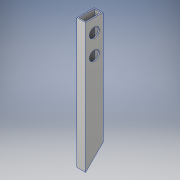
# Autodesk Inventor part: StorageSupport.ver1-1111-2020
Saved by Autodesk Inventor 2018 (Build 220112000, 112)
## iProperties
Created: 2020-01-25
Part Number: StorageSupport.ver1-1111-2020
Material: Aluminum 6061
Document SubType Name: Modeling
Designer: JMHal
Density: 2.7 g/cm^3
Appearance: Aluminum - Flat
Author: JMHal
Autodesk Inventor part; units mm, degrees
ref_plane "YZ Plane" through (0, 0, 0) normal (1, 0, 0) x (0, 1, 0)
ref_plane "XZ Plane" through (0, 0, 0) normal (0, 1, 0) x (-1, 0, 0)
ref_plane "XY Plane" through (0, 0, 0) normal (0, 0, 1) x (1, 0, 0)
sketch "Sketch1" plane through (0, 0, 0) normal (0, 1, 0) x (-1, 0, 0)
  line L0 (0, 0) -> (25.4, 0)
  line L1 (25.4, 0) -> (25.4, -50.8)
  line L2 (25.4, -50.8) -> (0, -50.8)
  line L3 (0, -50.8) -> (0, 0)
  line L4 (22.225, -3.175) -> (3.175, -3.175)
  line L5 (3.175, -3.175) -> (3.175, -47.625)
  line L6 (3.175, -47.625) -> (22.225, -47.625)
  line L7 (22.225, -47.625) -> (22.225, -3.175)
  dimension "d0" = 25.4
  dimension "d1" = 50.8
  dimension "d2" = 3.175
  constraints: 16 end point, 4 parallel, 2 perpendicular, 1 horizontal, 3 other
  measures "d0" distance of L1.end L2.end
  measures "d1" distance of L0.end L1.end
  measures "d2" distance between parallel lines of L0 L4
extrude "Extrusion1" add sketch "Sketch1" along normal blind 106.553
sketch "Sketch3" plane through (0, 0, 0) normal (1, 0, 0) x (0, 0, -1)
  line L0 (50.8, 0) -> (0, 0) projected
  line L1 (50.8, 0) -> (50.8, 106.553) projected
  line L2 (0, 106.553) -> (50.8, 106.553) projected
  line L3 (0, 0) -> (0, 106.553) projected
  point P0 (25.4, 68.453)
  dimension "d19" = 38.1
  measures "d19" distance from line of L2 point (25.4, 68.453)
hole "Hole2" at (0, 68.453, -25.4) direction (-1, 0, 0) diameter 28.575 end through all
sketch "Sketch4" plane through (0, 0, 0) normal (0, -1, 0) x (1, 0, 0)
  line L0 (-22.225, -47.625) -> (-22.225, -3.175) projected
  line L1 (-22.225, -3.175) -> (-3.175, -3.175) projected
  line L2 (-3.175, -3.175) -> (-3.175, -47.625) projected
  line L3 (-3.175, -47.625) -> (-22.225, -47.625) projected
  line L4 (0, 0) -> (-25.4, 0) projected
  line L5 (-25.4, 0) -> (-25.4, -50.8) projected
  line L6 (-25.4, -50.8) -> (0, -50.8) projected
  line L7 (0, -50.8) -> (0, 0) projected
extrude "Extrusion2" add sketch "Sketch4" along normal blind 254
sketch "Sketch5" plane through (0, 106.553, 0) normal (1, 0, 0) x (0, 0, -1)
  circle A0 centre (25.4, -38.1) radius 14.2875 projected
  line L0 (50.8, 0) -> (50.8, -360.553) projected
  line L1 (0, 0) -> (50.8, 0) projected
  line L2 (0, -360.553) -> (0, 0) projected
  line L3 (50.8, -360.553) -> (0, -360.553) projected
  line L4 (0, -360.553) -> (23.3209, -360.553)
  line L5 (0, -360.553) -> (50.8, -360.553) projected
  line L6 (0, -360.553) -> (9.2137, -369.7667)
  line L7 (0, -360.553) -> (9.2137, -360.553)
  line L8 (9.2137, -360.553) -> (9.2137, -369.7667)
  line L9 (9.2137, -369.7667) -> (0, -369.7667)
  line L10 (0, -369.7667) -> (0, -360.553)
  line L11 (0, -369.7667) -> (0, -378.9805)
  line L12 (0, -378.9805) -> (50.8, -328.1805)
  line L13 (50.8, 0) -> (50.8, -360.553) projected
  line L14 (50.8, -328.1805) -> (0, -328.1805)
  line L15 (0, -328.1805) -> (0, -378.9805)
  line L16 (0, -378.9805) -> (50.8, -378.9805)
  line L17 (50.8, -378.9805) -> (50.8, -328.1805)
  point P0 (0, -106.553)
  dimension "d22" = 13.0302
  dimension "d23" = 45
  dimension "d24" = 45
  constraints: 24 end point, 4 parallel, 3 horizontal, 2 perpendicular, 1 point on line, 1 vertical
  measures "d22" distance of L2.start L6.end
  measures "d23" angle of L3 L6
  measures "d24" angle of L3 L12
extrude "Extrusion3" add sketch "Sketch5" against normal blind 25.4 contours L12 L3 L2 L14 | L12 L8 L3 | L8 L6 L3 | L9 L10 L6 | L12 L11 L9
extrude "Extrusion4" cut sketch "Sketch5" against normal blind 25.4 contours L0 L3 L12 | L17 L16 L12 L3
sketch "Sketch6" plane through (0, 106.553, 0) normal (0, 1, 0) x (1, 0, 0)
  line L0 (-22.225, 3.175) -> (-22.225, 47.625) projected
  line L1 (-3.175, 3.175) -> (-22.225, 3.175) projected
  line L2 (-3.175, 47.625) -> (-3.175, 3.175) projected
  line L3 (-22.225, 47.625) -> (-3.175, 47.625) projected
  point P0 (0, 0)
extrude "Extrusion5" cut sketch "Sketch6" against normal through all
sketch "Sketch7" plane through (0, 106.553, 0) normal (1, 0, 0) x (0, 0, -1)
  line L0 (0, -378.9805) -> (50.8, -328.1805) projected
  line L1 (50.8, 0) -> (50.8, -328.1805) projected
  line L2 (0, 0) -> (50.8, 0) projected
  line L3 (0, -378.9805) -> (0, 0) projected
  circle A0 centre (25.4, -38.1) radius 14.2875 projected
  point P0 (0, -106.553)
  point P1 (25.4, -96.0374)
  dimension "d31" = 57.9374
  measures "d31" distance of point (25.4, -96.037) A0.centre
hole "Hole3" at (0, 10.5156, -25.4) direction (-1, 0, 0) diameter 28.575 end through all
body "Solid1"
